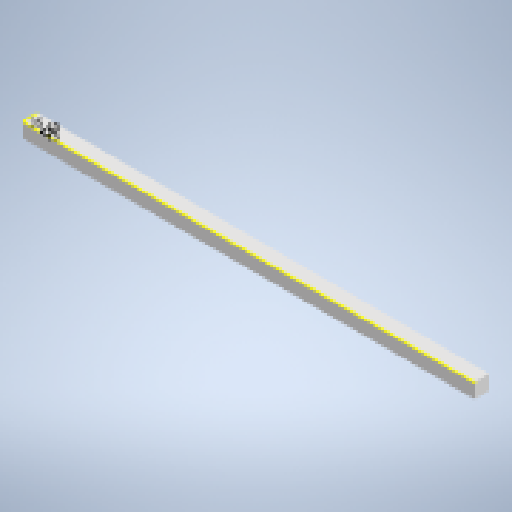
# Autodesk Inventor part: Nhom30
Saved by Autodesk Inventor 2023 (Build 270158000, 158)
## iProperties
Created: 2025-03-27
Part Number: Nhom30
Material: Generic
Document SubType Name: Modeling
Designer: huyqu
Density: 1 g/cm^3
Appearance: Default
Author: huyqu
Autodesk Inventor part; units mm, degrees
ref_plane "YZ Plane" through (0, 0, 0) normal (1, 0, 0) x (0, 1, 0)
ref_plane "XZ Plane" through (0, 0, 0) normal (0, 1, 0) x (-1, 0, 0)
ref_plane "XY Plane" through (0, 0, 0) normal (0, 0, 1) x (1, 0, 0)
sketch "Sketch1" plane through (0, 0, 0) normal (0, 0, 1) x (1, 0, 0)
  line L0 (0, 0) -> (920, 0)
  line L1 (920, 0) -> (920, 30)
  line L2 (920, 30) -> (0, 30)
  line L3 (0, 30) -> (0, 0)
  dimension "d0" = 30
  dimension "d1" = 920
  constraints: 8 end point, 2 parallel, 1 horizontal, 1 perpendicular
  measures "d0" distance between parallel lines of L0 L2
  measures "d1" distance of L1.end L2.end
extrude "Extrusion1" add sketch "Sketch1" along normal blind 30
sketch "Sketch2" plane through (0, 30, 0) normal (0, 1, 0) x (1, 0, 0)
  line L0 (920, -30) -> (0, -30) projected
  line L1 (50, -30) -> (65, -30)
  line L2 (65, -30) -> (65, -15)
  line L3 (65, -15) -> (50, -15)
  line L4 (50, -15) -> (50, -30)
  line L5 (0, 0) -> (0, -30) projected
  line L6 (870, -30) -> (855, -30)
  line L7 (855, -30) -> (855, -15)
  line L8 (855, -15) -> (870, -15)
  line L9 (870, -15) -> (870, -30)
  line L10 (920, 0) -> (920, -30) projected
  dimension "d4" = 15
  dimension "d5" = 15
  dimension "d6" = 50
  dimension "d7" = 15
  dimension "d8" = 15
  dimension "d9" = 50
  constraints: 16 end point, 4 parallel, 2 horizontal, 2 perpendicular, 2 point on line
  measures "d4" distance of L1.end L2.end
  measures "d5" distance of L2.end L3.end
  measures "d6" distance between parallel lines of L5 L4
  measures "d7" distance of L7.end L8.end
  measures "d8" distance of L6.end L7.end
  measures "d9" distance between parallel lines of L9 L10
extrude "Extrusion2" add sketch "Sketch2" along normal blind 1120
body "Solid1"
